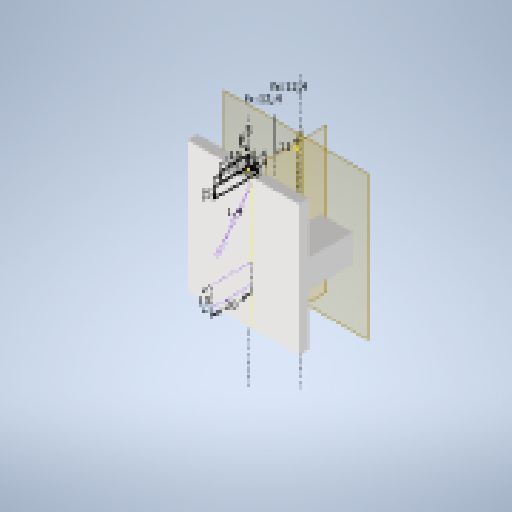
# Autodesk Inventor part: Backside
Saved by Autodesk Inventor 2023 (Build 270158000, 158)
## iProperties
Created: 2023-08-19
Part Number: Backside
Material: Generic
Document SubType Name: Modeling
Designer: Felix
Density: 1 g/cm^3
Appearance: Default
Author: Felix
Autodesk Inventor part; units mm, degrees
ref_plane "YZ Plane" through (0, 0, 0) normal (1, 0, 0) x (0, 1, 0)
ref_plane "XZ Plane" through (0, 0, 0) normal (0, 1, 0) x (-1, 0, 0)
ref_plane "XY Plane" through (0, 0, 0) normal (0, 0, 1) x (1, 0, 0)
ref_plane "Work Plane1" through (0, 0, 0) normal (0, 0, 1) x (1, 0, 0)
sketch "Sketch1" plane through (0, 0, 0) normal (0, 0, 1) x (1, 0, 0)
  circle A0 centre (49.6, -29.75) radius 2.55 construction
  circle A1 centre (9.9, -29.75) radius 3.6 construction
  circle A2 centre (49.9, -49.75) radius 11.95 projected
  circle A3 centre (49.9, -9.75) radius 11.95 projected
  circle A4 centre (9.9, -9.75) radius 11.95 projected
  circle A5 centre (9.9, -49.75) radius 11.95 projected
  line L0 (57.6, -22.75) -> (41.6, -22.75)
  line L1 (41.6, -22.75) -> (41.6, -36.75)
  line L2 (41.6, -36.75) -> (57.6, -36.75)
  line L3 (57.6, -36.75) -> (57.6, -22.75)
  line L4 (57.6, -22.75) -> (41.6, -36.75) construction
  line L5 (41.6, -22.75) -> (57.6, -36.75) construction
  line L6 (17.9, -22.75) -> (1.9, -22.75)
  line L7 (1.9, -22.75) -> (1.9, -36.75)
  line L8 (1.9, -36.75) -> (17.9, -36.75)
  line L9 (17.9, -36.75) -> (17.9, -22.75)
  line L10 (17.9, -22.75) -> (1.9, -36.75) construction
  line L11 (1.9, -22.75) -> (17.9, -36.75) construction
  circle A6 centre (9.9, -29.75) radius 2.65
  circle A7 centre (49.6, -29.75) radius 2.65
  point P0 (0, 0)
  dimension "d0" = 16
  dimension "d1" = 14
  dimension "d2" = 16
  dimension "d3" = 14
  dimension "d4" = 5.3
  dimension "d5" = 5.3
  constraints: 24 end point, 4 midpoint, 4 parallel, 2 centre point, 2 coincident, 2 horizontal, 2 perpendicular
  measures "d0" distance of L2.end L1.end
  measures "d1" distance of L1.end L0.end
  measures "d2" distance of L8.end L7.end
  measures "d3" distance of L7.end L6.end
  measures "d4" diameter of A6
  measures "d5" diameter of A7
extrude "Extrusion1" add sketch "Sketch1" along normal blind 22 contours L3 L2 L1 L0 | L9 L8 L7 L6
sketch "Sketch2" plane through (0, 0, 22) normal (0, 0, 1) x (1, 0, 0)
  line L0 (57.6, -36.75) -> (57.6, -22.75) construction
  line L1 (1.9, -22.75) -> (1.9, -36.75) construction
  line L2 (17.9, -36.75) -> (17.9, -22.75) construction
  line L3 (41.6, -22.75) -> (41.6, -36.75) construction
  line L4 (57.6, 3) -> (1.9, 3)
  line L5 (1.9, 3) -> (1.9, -62.5)
  line L6 (1.9, -62.5) -> (57.6, -62.5)
  line L7 (57.6, -62.5) -> (57.6, 3)
  line L8 (0, 3) -> (59.5, 3) construction
  line L9 (59.5, -62.5) -> (0, -62.5) construction
  point P0 (0, 0)
  constraints: 8 end point, 4 point on line, 2 parallel, 1 horizontal, 1 perpendicular
extrude "Extrusion2" add sketch "Sketch2" along normal blind 5
ref_plane "Work Plane2" through (29.75, -29.75, -3) normal (-1, 0, 0) x (0, 0, 1)
sketch "Sketch3" plane through (29.75, -29.75, -3) normal (-1, 0, 0) x (0, 0, 1)
  line L0 (0, 32.75) -> (3, 32.75) construction
  line L1 (0, -32.75) -> (3, -32.75) construction
  line L2 (14, 32.75) -> (14, -32.75) construction
  line L3 (3, 32.75) -> (3, -32.75) construction
  line L4 (26.4, 56.4687) -> (26.4, -62.1939) construction
  line L5 (1.6, 61.8459) -> (1.6, -76.3482) construction
  arc A0 (26.4, 39.15) -> (31.4, 34.15) centre (31.4, 39.15) ccw
  line L6 (25, 32.75) -> (30, 32.75) projected
  line L7 (25, -32.75) -> (30, -32.75) projected
  line L8 (26.4, 39.15) -> (31.4, 39.15)
  line L9 (31.4, 39.15) -> (41.4, 39.15)
  line L10 (41.4, 39.15) -> (41.4, 34.15)
  line L11 (41.4, 34.15) -> (31.4, 34.15)
  point P0 (3, 29.75)
  dimension "d10" = 11
  dimension "d11" = 12.4
  dimension "d12" = 12.4
  dimension "d13" = 5
  dimension "d14" = 1.4
  dimension "d15" = 15
  constraints: 16 end point, 2 parallel, 2 perpendicular, 2 point on circle, 2 point on line, 2 tangent, 2 vertical, 1 centre point, 1 horizontal
  measures "d10" distance between parallel lines of L3 L2
  measures "d11" distance between parallel lines of L5 L2
  measures "d12" distance between parallel lines of L4 L2
  measures "d13" radius of A0
  measures "d14" distance edge to line of A0 L6
  measures "d15" distance from line of L10 L8.start
ref_plane "Work Plane3" through (33.7, -29.75, -3) normal (1, 0, 0) x (0, 0, -1)
sketch "Sketch4" plane through (33.7, -29.75, -3) normal (1, 0, 0) x (0, 0, -1)
  arc A0 (-29.4, 32.75) -> (-26.4, 35.75) centre (-29.4, 35.75) ccw
  arc A1 (-26.4, 35.75) -> (-28.4, 37.75) centre (-28.4, 35.75) ccw
  line L0 (-29.4, 32.75) -> (-48.4, 32.75)
  line L1 (-48.4, 32.75) -> (-48.4, 37.75)
  line L2 (-48.4, 37.75) -> (-28.4, 37.75)
  line L3 (-30, -32.75) -> (-30, 32.75) construction
  line L4 (-25, 32.75) -> (-30, 32.75) construction
  line L5 (-25, 7) -> (-25, 32.75) construction
  line L6 (-27.0273, 33.9142) -> (-47.8508, 7) construction
  line L7 (-25.0481, 34.1845) -> (-46.9611, 5.8621) construction
  line L8 (-30, 32.75) -> (-30, -32.75) construction
  line L9 (-30, -4.418) -> (-50, -4.418) construction
  line L10 (-50, -4.418) -> (-50, -14.418) construction
  line L11 (-50, -14.418) -> (-30, -14.418) construction
  line L12 (-30, -14.418) -> (-30, -4.418) construction
  dimension "d16" = 3
  dimension "d17" = 2
  dimension "d19" = 3
  dimension "d20" = 5
  dimension "d21" = 20
  dimension "d22" = 1.4
  dimension "d23" = 1.4
  dimension "d24" = 20
  dimension "d25" = 10
  constraints: 18 end point, 6 point on circle, 4 parallel, 4 tangent, 2 centre point, 2 horizontal, 2 perpendicular, 2 point on line
  measures "d16" radius of A0
  measures "d17" radius of A1
  measures "d19" distance from line of L0 A0.end
  measures "d20" distance of L0.end L1.end
  measures "d21" distance of L1.end L2.end
  measures "d22" distance from line of L5 A0.end
  measures "d23" distance between parallel lines of L6 L7
  measures "d24" distance of L11.end L10.end
  measures "d25" distance of L10.end L9.end
equation "\"d3\" = d1"
equation "\"d4\" = d5"
equation "\"d12\" = d11"
equation "\"d19\" = d16"
body "Solid1"
